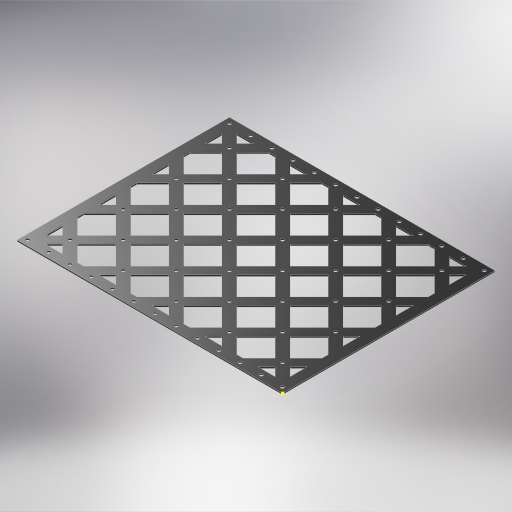
# Autodesk Inventor part: belly pan
Saved by Autodesk Inventor 2024 (Build 280153000, 153)
## iProperties
Created: 2023-12-20
Part Number: belly pan
Material: Generic
Document SubType Name: Modeling
Designer: elite
Density: 1 g/cm^3
Appearance: Glossy - Black
Author: elite
Autodesk Inventor part; units mm, degrees
ref_plane "YZ Plane" through (0, 0, 0) normal (1, 0, 0) x (0, 1, 0)
ref_plane "XZ Plane" through (0, 0, 0) normal (0, 1, 0) x (-1, 0, 0)
ref_plane "XY Plane" through (0, 0, 0) normal (0, 0, 1) x (1, 0, 0)
sketch "Sketch1" plane through (0, 0, 0) normal (0, 1, 0) x (-1, 0, 0)
  line L0 (0, 0) -> (317.5, 0)
  line L1 (317.5, 0) -> (317.5, -254)
  line L2 (317.5, -254) -> (0, -254)
  line L3 (0, -254) -> (0, 0)
  circle A0 centre (311.15, -6.35) radius 2.1082
  circle A1 centre (6.35, -6.35) radius 2.1082
  circle A2 centre (6.35, -247.65) radius 2.1082
  circle A3 centre (311.15, -247.65) radius 2.1082
  line L4 (304.8, -241.3) -> (12.7, -241.3)
  line L5 (12.7, -241.3) -> (12.7, -12.7)
  line L6 (12.7, -12.7) -> (304.8, -12.7)
  line L7 (304.8, -12.7) -> (304.8, -241.3)
  line L8 (304.8, -12.7) -> (76.2, -241.3)
  line L9 (304.8, -241.3) -> (76.2, -12.7)
  line L10 (12.7, -241.3) -> (241.3, -12.7)
  line L11 (6.35, -6.35) -> (241.3, -241.3)
  line L12 (295.8197, -12.7) -> (67.2197, -241.3)
  line L13 (304.8, -21.6803) -> (85.1803, -241.3)
  line L14 (304.8, -232.3197) -> (85.1803, -12.7)
  line L15 (295.8197, -241.3) -> (67.2197, -12.7)
  line L16 (10.8401, -1.8599) -> (250.2803, -241.3)
  line L17 (1.8599, -10.8401) -> (232.3197, -241.3)
  line L18 (12.7, -232.3197) -> (232.3197, -12.7)
  line L19 (21.6803, -241.3) -> (250.2803, -12.7)
  line L20 (368.3, -241.3) -> (139.7, -12.7)
  line L21 (359.3197, -241.3) -> (130.7197, -12.7)
  line L22 (368.3, -232.3197) -> (148.6803, -12.7)
  line L23 (431.8, -241.3) -> (203.2, -12.7)
  line L24 (422.8197, -241.3) -> (194.2197, -12.7)
  line L25 (431.8, -232.3197) -> (212.1803, -12.7)
  line L26 (495.3, -241.3) -> (266.7, -12.7)
  line L27 (486.3197, -241.3) -> (257.7197, -12.7)
  line L28 (495.3, -232.3197) -> (275.6803, -12.7)
  line L29 (241.3, -241.3) -> (12.7, -12.7)
  line L30 (232.3197, -241.3) -> (3.7197, -12.7)
  line L31 (241.3, -232.3197) -> (21.6803, -12.7)
  line L32 (304.8, -241.3) -> (76.2, -12.7)
  line L33 (295.8197, -241.3) -> (67.2197, -12.7)
  line L34 (304.8, -232.3197) -> (85.1803, -12.7)
  line L35 (368.3, -241.3) -> (139.7, -12.7)
  line L36 (359.3197, -241.3) -> (130.7197, -12.7)
  line L37 (368.3, -232.3197) -> (148.6803, -12.7)
  line L38 (431.8, -241.3) -> (203.2, -12.7)
  line L39 (422.8197, -241.3) -> (194.2197, -12.7)
  line L40 (431.8, -232.3197) -> (212.1803, -12.7)
  line L41 (177.8, -241.3) -> (-50.8, -12.7)
  line L42 (168.8197, -241.3) -> (-59.7803, -12.7)
  line L43 (177.8, -232.3197) -> (-41.8197, -12.7)
  line L44 (241.3, -241.3) -> (12.7, -12.7)
  line L45 (232.3197, -241.3) -> (3.7197, -12.7)
  line L46 (241.3, -232.3197) -> (21.6803, -12.7)
  line L47 (304.8, -241.3) -> (76.2, -12.7)
  line L48 (295.8197, -241.3) -> (67.2197, -12.7)
  line L49 (304.8, -232.3197) -> (85.1803, -12.7)
  line L50 (368.3, -241.3) -> (139.7, -12.7)
  line L51 (359.3197, -241.3) -> (130.7197, -12.7)
  line L52 (368.3, -232.3197) -> (148.6803, -12.7)
  line L53 (114.3, -241.3) -> (-114.3, -12.7)
  line L54 (105.3197, -241.3) -> (-123.2803, -12.7)
  line L55 (114.3, -232.3197) -> (-105.3197, -12.7)
  line L56 (177.8, -241.3) -> (-50.8, -12.7)
  line L57 (168.8197, -241.3) -> (-59.7803, -12.7)
  line L58 (177.8, -232.3197) -> (-41.8197, -12.7)
  line L59 (241.3, -241.3) -> (12.7, -12.7)
  line L60 (232.3197, -241.3) -> (3.7197, -12.7)
  line L61 (241.3, -232.3197) -> (21.6803, -12.7)
  line L62 (304.8, -241.3) -> (76.2, -12.7)
  line L63 (295.8197, -241.3) -> (67.2197, -12.7)
  line L64 (304.8, -232.3197) -> (85.1803, -12.7)
  line L65 (50.8, -241.3) -> (-177.8, -12.7)
  line L66 (41.8197, -241.3) -> (-186.7803, -12.7)
  line L67 (50.8, -232.3197) -> (-168.8197, -12.7)
  line L68 (114.3, -241.3) -> (-114.3, -12.7)
  line L69 (105.3197, -241.3) -> (-123.2803, -12.7)
  line L70 (114.3, -232.3197) -> (-105.3197, -12.7)
  line L71 (177.8, -241.3) -> (-50.8, -12.7)
  line L72 (168.8197, -241.3) -> (-59.7803, -12.7)
  line L73 (177.8, -232.3197) -> (-41.8197, -12.7)
  line L74 (241.3, -241.3) -> (12.7, -12.7)
  line L75 (232.3197, -241.3) -> (3.7197, -12.7)
  line L76 (241.3, -232.3197) -> (21.6803, -12.7)
  line L77 (177.8, -232.3197) -> (186.7803, -241.3)
  line L78 (114.3, -232.3197) -> (123.2803, -241.3)
  line L79 (50.8, -232.3197) -> (59.7803, -241.3)
  line L80 (85.1803, -241.3) -> (313.7803, -12.7)
  line L81 (76.2, -232.3197) -> (295.8197, -12.7)
  line L82 (76.2, -241.3) -> (304.8, -12.7)
  line L83 (148.6803, -241.3) -> (377.2803, -12.7)
  line L84 (139.7, -232.3197) -> (359.3197, -12.7)
  line L85 (139.7, -241.3) -> (368.3, -12.7)
  line L86 (212.1803, -241.3) -> (440.7803, -12.7)
  line L87 (203.2, -232.3197) -> (422.8197, -12.7)
  line L88 (203.2, -241.3) -> (431.8, -12.7)
  line L89 (275.6803, -241.3) -> (504.2803, -12.7)
  line L90 (266.7, -232.3197) -> (486.3197, -12.7)
  line L91 (266.7, -241.3) -> (495.3, -12.7)
  line L92 (-41.8197, -241.3) -> (186.7803, -12.7)
  line L93 (-50.8, -232.3197) -> (168.8197, -12.7)
  line L94 (-50.8, -241.3) -> (177.8, -12.7)
  line L95 (21.6803, -241.3) -> (250.2803, -12.7)
  line L96 (12.7, -232.3197) -> (232.3197, -12.7)
  line L97 (12.7, -241.3) -> (241.3, -12.7)
  line L98 (85.1803, -241.3) -> (313.7803, -12.7)
  line L99 (76.2, -232.3197) -> (295.8197, -12.7)
  line L100 (76.2, -241.3) -> (304.8, -12.7)
  line L101 (148.6803, -241.3) -> (377.2803, -12.7)
  line L102 (139.7, -232.3197) -> (359.3197, -12.7)
  line L103 (139.7, -241.3) -> (368.3, -12.7)
  line L104 (212.1803, -241.3) -> (440.7803, -12.7)
  line L105 (203.2, -232.3197) -> (422.8197, -12.7)
  line L106 (203.2, -241.3) -> (431.8, -12.7)
  line L107 (-105.3197, -241.3) -> (123.2803, -12.7)
  line L108 (-114.3, -232.3197) -> (105.3197, -12.7)
  line L109 (-114.3, -241.3) -> (114.3, -12.7)
  line L110 (-41.8197, -241.3) -> (186.7803, -12.7)
  line L111 (-50.8, -232.3197) -> (168.8197, -12.7)
  line L112 (-50.8, -241.3) -> (177.8, -12.7)
  line L113 (21.6803, -241.3) -> (250.2803, -12.7)
  line L114 (12.7, -232.3197) -> (232.3197, -12.7)
  line L115 (12.7, -241.3) -> (241.3, -12.7)
  line L116 (85.1803, -241.3) -> (313.7803, -12.7)
  line L117 (76.2, -232.3197) -> (295.8197, -12.7)
  line L118 (76.2, -241.3) -> (304.8, -12.7)
  line L119 (148.6803, -241.3) -> (377.2803, -12.7)
  line L120 (139.7, -232.3197) -> (359.3197, -12.7)
  line L121 (139.7, -241.3) -> (368.3, -12.7)
  line L122 (-168.8197, -241.3) -> (59.7803, -12.7)
  line L123 (-177.8, -232.3197) -> (41.8197, -12.7)
  line L124 (-177.8, -241.3) -> (50.8, -12.7)
  line L125 (-105.3197, -241.3) -> (123.2803, -12.7)
  line L126 (-114.3, -232.3197) -> (105.3197, -12.7)
  line L127 (-114.3, -241.3) -> (114.3, -12.7)
  line L128 (-41.8197, -241.3) -> (186.7803, -12.7)
  line L129 (-50.8, -232.3197) -> (168.8197, -12.7)
  line L130 (-50.8, -241.3) -> (177.8, -12.7)
  line L131 (21.6803, -241.3) -> (250.2803, -12.7)
  line L132 (12.7, -232.3197) -> (232.3197, -12.7)
  line L133 (12.7, -241.3) -> (241.3, -12.7)
  line L134 (85.1803, -241.3) -> (313.7803, -12.7)
  line L135 (76.2, -232.3197) -> (295.8197, -12.7)
  line L136 (76.2, -241.3) -> (304.8, -12.7)
  line L137 (139.7, -232.3197) -> (130.7197, -241.3)
  line L138 (203.2, -232.3197) -> (194.2197, -241.3)
  line L139 (266.7, -232.3197) -> (257.7197, -241.3)
  point P0 (304.8, -59.7803)
  point P1 (257.7197, -12.7)
  point P2 (276.7697, -31.75)
  point P3 (254, -54.5197)
  point P4 (262.9803, -63.5)
  point P5 (285.75, -40.7303)
  point P6 (285.75, -22.7697)
  point P7 (275.6803, -12.7)
  point P8 (304.8, -41.8197)
  point P9 (294.7303, -31.75)
  point P10 (231.2303, -95.25)
  point P11 (254, -72.4803)
  point P12 (276.7697, -95.25)
  point P13 (254, -118.0197)
  point P14 (222.25, -104.2303)
  point P15 (245.0197, -127)
  point P16 (222.25, -149.7697)
  point P17 (226.7401, -154.2599)
  point P18 (249.5099, -131.4901)
  point P19 (276.7697, -158.75)
  point P20 (254, -181.5197)
  point P21 (258.4901, -186.0099)
  point P22 (281.2599, -163.2401)
  point P23 (304.8, -186.7803)
  point P24 (304.8, -168.8197)
  point P25 (294.7303, -158.75)
  point P26 (304.8, -148.6803)
  point P27 (304.8, -130.7197)
  point P28 (285.75, -149.7697)
  point P29 (262.9803, -127)
  point P30 (285.75, -104.2303)
  point P31 (304.8, -123.2803)
  point P32 (304.8, -105.3197)
  point P33 (294.7303, -95.25)
  point P34 (304.8, -85.1803)
  point P35 (304.8, -67.2197)
  point P36 (285.75, -86.2697)
  point P37 (231.2303, -31.75)
  point P38 (222.25, -22.7697)
  point P39 (212.1803, -12.7)
  point P40 (194.2197, -12.7)
  point P41 (213.2697, -31.75)
  point P42 (190.5, -54.5197)
  point P43 (167.7303, -31.75)
  point P44 (186.7803, -12.7)
  point P45 (168.8197, -12.7)
  point P46 (158.75, -22.7697)
  point P47 (148.6803, -12.7)
  point P48 (130.7197, -12.7)
  point P49 (213.2697, -95.25)
  point P50 (190.5, -118.0197)
  point P51 (199.4803, -127)
  point P52 (222.25, -86.2697)
  point P53 (199.4803, -63.5)
  point P54 (222.25, -40.7303)
  point P55 (245.0197, -63.5)
  point P56 (222.25, -167.7303)
  point P57 (245.0197, -190.5)
  point P58 (222.25, -213.2697)
  point P59 (199.4803, -190.5)
  point P60 (158.75, -231.2303)
  point P61 (167.7303, -222.25)
  point P62 (190.5, -199.4803)
  point P63 (213.2697, -222.25)
  point P64 (222.25, -231.2303)
  point P65 (231.2303, -222.25)
  point P66 (254, -199.4803)
  point P67 (276.7697, -222.25)
  point P68 (285.75, -231.2303)
  point P69 (294.7303, -222.25)
  point P70 (304.8, -212.1803)
  point P71 (304.8, -194.2197)
  point P72 (285.75, -213.2697)
  point P73 (262.9803, -190.5)
  point P74 (285.75, -167.7303)
  point P75 (231.2303, -158.75)
  point P76 (254, -135.9803)
  point P77 (40.7303, -222.25)
  point P78 (31.75, -231.2303)
  point P79 (190.5, -135.9803)
  point P80 (213.2697, -158.75)
  point P81 (167.7303, -95.25)
  point P82 (158.75, -104.2303)
  point P83 (181.5197, -127)
  point P84 (158.75, -149.7697)
  point P85 (135.9803, -127)
  point P86 (127, -135.9803)
  point P87 (149.7697, -158.75)
  point P88 (127, -181.5197)
  point P89 (104.2303, -158.75)
  point P90 (95.25, -167.7303)
  point P91 (118.0197, -190.5)
  point P92 (95.25, -213.2697)
  point P93 (72.4803, -190.5)
  point P94 (63.5, -199.4803)
  point P95 (86.2697, -222.25)
  point P96 (95.25, -231.2303)
  point P97 (104.2303, -222.25)
  point P98 (127, -199.4803)
  point P99 (149.7697, -222.25)
  point P100 (158.75, -213.2697)
  point P101 (135.9803, -190.5)
  point P102 (158.75, -167.7303)
  point P103 (181.5197, -190.5)
  point P104 (190.5, -181.5197)
  point P105 (167.7303, -158.75)
  point P106 (158.75, -86.2697)
  point P107 (135.9803, -63.5)
  point P108 (127, -72.4803)
  point P109 (149.7697, -95.25)
  point P110 (127, -118.0197)
  point P111 (104.2303, -95.25)
  point P112 (95.25, -104.2303)
  point P113 (118.0197, -127)
  point P114 (95.25, -149.7697)
  point P115 (72.4803, -127)
  point P116 (63.5, -135.9803)
  point P117 (86.2697, -158.75)
  point P118 (63.5, -181.5197)
  point P119 (40.7303, -158.75)
  point P120 (31.75, -167.7303)
  point P121 (54.5197, -190.5)
  point P122 (31.75, -213.2697)
  point P123 (12.7, -194.2197)
  point P124 (12.7, -212.1803)
  point P125 (22.7697, -222.25)
  point P126 (190.5, -72.4803)
  point P127 (181.5197, -63.5)
  point P128 (86.2697, -95.25)
  point P129 (63.5, -118.0197)
  point P130 (40.7303, -95.25)
  point P131 (63.5, -72.4803)
  point P132 (118.0197, -63.5)
  point P133 (95.25, -86.2697)
  point P134 (72.4803, -63.5)
  point P135 (95.25, -40.7303)
  point P136 (158.75, -40.7303)
  point P137 (149.7697, -31.75)
  point P138 (127, -54.5197)
  point P139 (104.2303, -31.75)
  point P140 (123.2803, -12.7)
  point P141 (105.3197, -12.7)
  point P142 (95.25, -22.7697)
  point P143 (86.2697, -31.75)
  point P144 (63.5, -54.5197)
  point P145 (40.7303, -31.75)
  point P146 (59.7803, -12.7)
  point P147 (41.8197, -12.7)
  point P148 (31.75, -22.7697)
  point P149 (21.6803, -12.7)
  point P150 (12.7, -21.6803)
  point P151 (22.7697, -31.75)
  point P152 (12.7, -41.8197)
  point P153 (12.7, -59.7803)
  point P154 (31.75, -40.7303)
  point P155 (54.5197, -63.5)
  point P156 (31.75, -86.2697)
  point P157 (12.7, -67.2197)
  point P158 (12.7, -85.1803)
  point P159 (22.7697, -95.25)
  point P160 (12.7, -105.3197)
  point P161 (12.7, -123.2803)
  point P162 (31.75, -104.2303)
  point P163 (54.5197, -127)
  point P164 (31.75, -149.7697)
  point P165 (12.7, -130.7197)
  point P166 (12.7, -148.6803)
  point P167 (22.7697, -158.75)
  point P168 (12.7, -168.8197)
  point P169 (12.7, -186.7803)
  dimension "d60" = 317.5
  dimension "d61" = 254
  dimension "d62" = 4.2164
  dimension "d63" = 6.35
  dimension "d64" = 6.35
  dimension "d65" = 4.2164
  dimension "d66" = 6.35
  dimension "d69" = 241.3
  dimension "d74" = 6.35
  dimension "d75" = 12.7
  dimension "d76" = 12.7
  dimension "d77" = 12.7
  dimension "d78" = 12.7
  dimension "d79" = 45
  dimension "d80" = 45
  dimension "d81" = 45
  dimension "d82" = 45
  dimension "d83" = 6.35
  dimension "d84" = 6.35
  dimension "d85" = 6.35
  dimension "d86" = 6.35
  dimension "d87" = 6.35
  dimension "d88" = 6.35
  dimension "d89" = 6.35
  dimension "d90" = 6.35
  dimension "d93" = 63.5
  dimension "d96" = 63.5
  dimension "d101" = 63.5
  dimension "d104" = 63.5
  constraints: 276 end point, 228 horizontal alignment, 128 parallel, 4 centre point, 4 point on line, 2 vertical, 1 horizontal, 1 perpendicular, 30 other
  measures "d60" distance of L1.end L2.end
  measures "d61" distance of L0.end L1.end
  measures "d62" diameter of A0
  measures "d63" distance from line of L0 A0.centre
  measures "d64" distance from line of L1 A0.centre
  measures "d65" diameter of A1
  measures "d66" distance from line of L3 L11.start
  measures "d69" distance of L11.start A2.centre
  measures "d74" distance from line of L0 L11.start
  measures "d76" distance between parallel lines of L1 L7
  measures "d78" distance between parallel lines of L3 L5
  measures "d79" angle to the sketch x axis of L8
  measures "d80" angle of L7 L9
  measures "d81" angle of L5 L10
  measures "d82" angle of L5 L11
  measures "d83" distance between parallel lines of L8 L12
  measures "d84" distance between parallel lines of L8 L13
  measures "d85" distance between parallel lines of L9 L14
  measures "d86" distance between parallel lines of L9 L15
  measures "d87" distance between parallel lines of L11 L16
  measures "d88" distance between parallel lines of L11 L17
  measures "d89" distance between parallel lines of L10 L18
  measures "d90" distance between parallel lines of L10 L19
  measures "d93" distance of L7.end L20.start
  measures "d96" distance of L7.end L29.start
  measures "d101" distance of L19.start L80.start
  measures "d104" distance of L19.start L92.start
extrude "Extrusion1" add sketch "Sketch1" along normal blind 1.5875 contours L0 L1 L28 L7 L6 L5 L123 L3 | L43 L124 L3 | L123 L5 L124 L43 | L84 L26 L7 L28 | L1 L26 L84 | L41 L122 L3 | L124 L43 L122 L41 | L124 L5 L122 L43 | L123 L17 L124 L5 | L85 L27 L84 L26 | L1 L27 L85 | L7 L26 L13 L28 | L84 L27 L7 L26 | L42 L5 L108 L3 | L122 L41 L5 L42 | L122 L43 L5 L41 | L122 L5 L43 | L124 L17 L122 L5 | L5 L11 L123 L17 | L123 L11 L124 L17 | L83 L7 L85 L27 | L1 L25 L7 L83 | L85 L7 L84 L27 | L13 L28 L8 L7 | L7 L27 L13 L26 | L13 L26 L8 L28 | L84 L7 L27 | L55 L109 L3 | L108 L5 L109 L55 | L5 L41 L108 L42 | L5 L43 L108 L41 | L124 L11 L122 L17 | L6 L16 L123 L11 | L123 L16 L124 L11 | L87 L23 L7 L25 | L1 L23 L87 | L83 L25 L85 L7 | L85 L25 L84 L7 | L8 L28 L12 L6 | L13 L27 L8 L26 | L8 L26 L12 L28 | L53 L107 L3 | L109 L55 L107 L53 | L109 L5 L107 L55 | L108 L42 L109 L5 | L108 L41 L109 L42 | L108 L43 L109 L41 | L108 L17 L109 L43 | L122 L11 L108 L17 | L124 L16 L122 L11 | L123 L6 L124 L16 | L88 L24 L87 L23 | L1 L24 L88 | L7 L23 L83 L25 | L87 L24 L7 L23 | L83 L23 L85 L25 | L85 L23 L84 L25 | L13 L25 L8 L27 | L8 L27 L12 L26 | L12 L26 L6 L28 | L84 L23 L13 L25 | L54 L5 L93 L3 | L107 L53 L5 L54 | L107 L55 L5 L53 | L107 L5 L55 | L109 L42 L107 L5 | L109 L41 L107 L42 | L109 L43 L107 L41 | L109 L17 L107 L43 | L108 L11 L109 L17 | L122 L16 L108 L11 | L124 L6 L122 L16 | L86 L7 L88 L24 | L1 L22 L7 L86 | L88 L7 L87 L24 | L7 L24 L83 L23 | L87 L7 L24 | L83 L24 L85 L23 | L85 L24 L84 L23 | L13 L23 L8 L25 | L8 L25 L12 L27 | L12 L27 L6 L26 | L84 L24 L13 L23 | L67 L94 L3 | L93 L5 L94 L67 | L5 L53 L93 L54 | L5 L55 L93 L53 | L107 L41 L93 L42 | L107 L43 L93 L41 | L109 L11 L107 L17 | L108 L16 L109 L11 | L90 L20 L7 L22 | L1 L20 L90 | L86 L22 L88 L7 | L88 L22 L87 L7 | L83 L22 L85 L24 | L85 L22 L84 L24 | L13 L24 L8 L23 | L8 L23 L12 L25 | L65 L92 L3 | L94 L67 L92 L65 | L94 L5 L92 L67 | L93 L54 L94 L5 | L93 L53 L94 L54 | L93 L55 L94 L53 | L93 L42 L94 L55 | L93 L41 L94 L42 | L93 L43 L94 L41 | L93 L17 L94 L43 | L107 L11 L93 L17 | L109 L16 L107 L11 | L108 L15 L109 L16 | L91 L21 L90 L20 | L1 L21 L91 | L7 L20 L86 L22 | L90 L21 L7 L20 | L86 L20 L88 L22 | L88 L20 L87 L22 | L87 L20 L83 L22 | L83 L20 L85 L22 | L85 L20 L84 L22 | L13 L22 L8 L24 | L8 L24 L12 L23 | L12 L23 L19 L25 | L84 L20 L13 L22 | L66 L5 L4 L7 L89 L1 L2 L3 | L92 L65 L5 L66 | L92 L67 L5 L65 | L92 L5 L67 | L94 L54 L92 L5 | L94 L53 L92 L54 | L94 L55 L92 L53 | L94 L42 L92 L55 | L94 L41 L92 L42 | L94 L43 L92 L41 | L94 L17 L92 L43 | L93 L11 L94 L17 | L107 L16 L93 L11 | L109 L15 L107 L16 | L108 L9 L109 L15 | L15 L6 L9 L108 | L89 L7 L91 L21 | L91 L7 L90 L21 | L7 L21 L86 L20 | L90 L7 L21 | L86 L21 L88 L20 | L88 L21 L87 L20 | L87 L21 L83 L20 | L83 L21 L85 L20 | L85 L21 L84 L20 | L19 L25 L10 L6 | L13 L20 L8 L22 | L8 L22 L12 L24 | L12 L24 L19 L23 | L19 L23 L10 L25 | L84 L21 L13 L20 | L5 L65 L18 L66 | L5 L67 L18 L65 | L92 L53 L18 L54 | L92 L55 L18 L53 | L92 L41 L18 L42 | L92 L43 L18 L41 | L94 L11 L92 L17 | L93 L16 L94 L11 | L109 L9 L107 L15 | L108 L14 L109 L9 | L9 L6 L14 L108 | L89 L14 L91 L7 | L91 L14 L90 L7 | L86 L14 L88 L21 | L88 L14 L87 L21 | L83 L14 L85 L21 | L85 L14 L84 L21 | L10 L25 L18 L6 | L13 L21 L8 L20 | L8 L20 L12 L22 | L19 L24 L10 L23 | L10 L23 L18 L25 | L18 L66 L10 L5 | L18 L65 L10 L66 | L18 L67 L10 L65 | L18 L54 L10 L67 | L18 L53 L10 L54 | L18 L55 L10 L53 | L18 L42 L10 L55 | L18 L41 L10 L42 | L18 L43 L10 L41 | L18 L17 L10 L43 | L92 L11 L18 L17 | L94 L16 L92 L11 | L93 L15 L94 L16 | L107 L9 L93 L15 | L109 L14 L107 L9 | L108 L6 L109 L14 | L7 L9 L89 L14 | L89 L9 L91 L14 | L91 L9 L90 L14 | L90 L9 L86 L14 | L86 L9 L88 L14 | L88 L9 L87 L14 | L87 L9 L83 L14 | L83 L9 L85 L14 | L85 L9 L84 L14 | L13 L14 L8 L21 | L8 L21 L12 L20 | L12 L20 L19 L22 | L19 L22 L10 L24 | L10 L24 L18 L23 | L18 L23 L6 L25 | L84 L9 L13 L14 | L10 L66 L19 L4 | L10 L65 L19 L66 | L10 L67 L19 L65 | L10 L54 L19 L67 | L10 L53 L19 L54 | L10 L55 L19 L53 | L10 L42 L19 L55 | L10 L41 L19 L42 | L10 L43 L19 L41 | L18 L11 L10 L17 | L10 L17 L19 L43 | L92 L16 L18 L11 | L94 L15 L92 L16 | L93 L9 L94 L15 | L107 L14 L93 L9 | L109 L6 L107 L14 | L4 L15 L89 L9 | L89 L15 L91 L9 | L91 L15 L90 L9 | L90 L15 L86 L9 | L86 L15 L88 L9 | L88 L15 L87 L9 | L87 L15 L83 L9 | L83 L15 L85 L9 | L85 L15 L84 L9 | L13 L9 L8 L14 | L8 L14 L12 L21 | L12 L21 L19 L20 | L19 L20 L10 L22 | L10 L22 L18 L24 | L18 L24 L6 L23 | L84 L15 L13 L9 | L19 L65 L4 L66 | L19 L67 L79 L4 L65 | L19 L53 L12 L54 | L19 L55 L12 L53 | L19 L41 L12 L42 | L19 L43 L12 L41 | L10 L11 L19 L17 | L18 L16 L10 L11 | L94 L9 L92 L15 | L93 L14 L94 L9 | L89 L4 L91 L15 | L91 L4 L139 L90 L15 | L86 L16 L88 L15 | L88 L16 L87 L15 | L83 L16 L85 L15 | L85 L16 L84 L15 | L13 L15 L8 L9 | L8 L9 L12 L14 | L19 L21 L10 L20 | L10 L20 L18 L22 | L54 L8 L4 L12 | L12 L53 L8 L54 | L12 L55 L8 L53 | L12 L42 L8 L55 | L12 L41 L8 L42 | L12 L43 L8 L41 | L10 L16 L19 L11 | L19 L11 L12 L17 | L18 L15 L10 L16 | L12 L17 L8 L43 | L92 L9 L18 L15 | L94 L14 L92 L9 | L93 L21 L94 L14 | L86 L11 L88 L16 | L16 L4 L11 L86 | L88 L11 L87 L16 | L87 L11 L83 L16 | L83 L11 L85 L16 | L85 L11 L84 L16 | L8 L15 L12 L9 | L13 L16 L8 L15 | L12 L9 L19 L14 | L19 L14 L10 L21 | L10 L21 L18 L20 | L18 L20 L92 L22 | L84 L11 L13 L16 | L54 L13 L4 L8 | L8 L53 L13 L54 | L8 L55 L13 L53 | L8 L42 L13 L55 | L8 L41 L13 L42 | L8 L43 L13 L41 | L10 L15 L19 L16 | L19 L16 L12 L11 | L12 L11 L8 L17 | L18 L9 L10 L15 | L8 L17 L13 L43 | L92 L14 L18 L9 | L94 L21 L92 L14 | L93 L20 L94 L21 | L21 L6 L20 L93 | L86 L17 L88 L11 | L11 L4 L17 L86 | L88 L17 L87 L11 | L87 L17 L83 L11 | L83 L17 L85 L11 | L85 L17 L84 L11 | L92 L22 L94 L6 | L8 L16 L12 L15 | L12 L15 L19 L9 | L13 L11 L8 L16 | L19 L9 L10 L14 | L10 L14 L18 L21 | L18 L21 L92 L20 | L92 L20 L94 L22 | L84 L17 L13 L11 | L13 L53 L4 L54 | L13 L55 L78 L4 L53 | L13 L41 L84 L42 | L13 L43 L84 L41 | L10 L9 L19 L15 | L12 L16 L8 L11 | L8 L11 L13 L17 | L18 L14 L10 L9 | L94 L20 L92 L21 | L93 L22 L94 L20 | L20 L6 L22 L93 | L86 L4 L88 L17 | L88 L4 L138 L87 L17 | L83 L43 L85 L17 | L85 L43 L84 L17 | L94 L22 L93 L6 | L84 L41 L85 L42 | L42 L85 L4 L137 L84 | L84 L43 L85 L41 | L83 L41 L85 L43 | L43 L77 L4 L41 L83 | L85 L41 L83 L42 | L42 L83 L4 L85 | L41 L4 L42 L83
sketch "Sketch3" plane through (0, 1.5875, 0) normal (0, 1, 0) x (1, 0, 0)
  circle A0 centre (-311.15, 6.35) radius 2.1082 projected
  line L0 (-317.5, 0) -> (0, 0) projected
  circle A1 centre (-311.15, 247.65) radius 2.1082 projected
  line L1 (0, 254) -> (-317.5, 254) projected
  circle A2 centre (-311.15, 247.65) radius 2.1082
  circle A3 centre (-311.15, 6.35) radius 2.1082
  circle A4 centre (-285.75, 6.35) radius 2.1082
  circle A5 centre (-285.75, 247.65) radius 2.1082
  circle A6 centre (-260.35, 6.35) radius 2.1082
  circle A7 centre (-260.35, 247.65) radius 2.1082
  circle A8 centre (-234.95, 6.35) radius 2.1082
  circle A9 centre (-234.95, 247.65) radius 2.1082
  circle A10 centre (-209.55, 6.35) radius 2.1082
  circle A11 centre (-209.55, 247.65) radius 2.1082
  circle A12 centre (-184.15, 6.35) radius 2.1082
  circle A13 centre (-184.15, 247.65) radius 2.1082
  circle A14 centre (-158.75, 6.35) radius 2.1082
  circle A15 centre (-158.75, 247.65) radius 2.1082
  circle A16 centre (-133.35, 6.35) radius 2.1082
  circle A17 centre (-133.35, 247.65) radius 2.1082
  circle A18 centre (-107.95, 6.35) radius 2.1082
  circle A19 centre (-107.95, 247.65) radius 2.1082
  circle A20 centre (-82.55, 6.35) radius 2.1082
  circle A21 centre (-82.55, 247.65) radius 2.1082
  circle A22 centre (-57.15, 6.35) radius 2.1082
  circle A23 centre (-57.15, 247.65) radius 2.1082
  circle A24 centre (-31.75, 6.35) radius 2.1082
  circle A25 centre (-31.75, 247.65) radius 2.1082
  circle A26 centre (-6.35, 6.35) radius 2.1082
  circle A27 centre (-6.35, 247.65) radius 2.1082
  circle A28 centre (19.05, 6.35) radius 2.1082
  circle A29 centre (19.05, 247.65) radius 2.1082
  dimension "d109" = 25.4
  constraints: 28 centre point, 2 coincident, 2 concentric, 1 horizontal, 52 other
  measures "d109" distance of A3.centre A4.centre
extrude "Extrusion3" cut sketch "Sketch3" against normal blind 317.5
sketch "Sketch4" plane through (0, 1.5875, 0) normal (0, 1, 0) x (1, 0, 0)
  point P0 (0, 0)
sketch "Sketch5" plane through (0, 1.5875, 0) normal (0, 1, 0) x (1, 0, 0)
  line L0 (-285.75, 22.7697) -> (-275.6803, 12.7) projected
  line L1 (-285.75, 40.7303) -> (-285.75, 22.7697)
  circle A0 centre (-285.75, 31.75) radius 2.1082
  line L2 (-317.5, 254) -> (-317.5, 0) projected
  line L3 (-317.5, 0) -> (0, 0) projected
  circle A1 centre (-222.25, 31.75) radius 2.1082
  circle A2 centre (-158.75, 31.75) radius 2.1082
  circle A3 centre (-95.25, 31.75) radius 2.1082
  circle A4 centre (-31.75, 31.75) radius 2.1082
  circle A5 centre (-285.75, 95.25) radius 2.1082
  circle A6 centre (-222.25, 95.25) radius 2.1082
  circle A7 centre (-158.75, 95.25) radius 2.1082
  circle A8 centre (-95.25, 95.25) radius 2.1082
  circle A9 centre (-31.75, 95.25) radius 2.1082
  circle A10 centre (-285.75, 158.75) radius 2.1082
  circle A11 centre (-222.25, 158.75) radius 2.1082
  circle A12 centre (-158.75, 158.75) radius 2.1082
  circle A13 centre (-95.25, 158.75) radius 2.1082
  circle A14 centre (-31.75, 158.75) radius 2.1082
  circle A15 centre (-285.75, 222.25) radius 2.1082
  circle A16 centre (-222.25, 222.25) radius 2.1082
  circle A17 centre (-158.75, 222.25) radius 2.1082
  circle A18 centre (-95.25, 222.25) radius 2.1082
  circle A19 centre (-31.75, 222.25) radius 2.1082
  line L4 (-254, 199.4803) -> (-254, 181.5197)
  circle A20 centre (-254, 190.5) radius 2.1082
  circle A21 centre (-254, 127) radius 2.1082
  circle A22 centre (-254, 63.5) radius 2.1082
  circle A23 centre (-190.5, 190.5) radius 2.1082
  circle A24 centre (-190.5, 127) radius 2.1082
  circle A25 centre (-190.5, 63.5) radius 2.1082
  circle A26 centre (-127, 190.5) radius 2.1082
  circle A27 centre (-127, 127) radius 2.1082
  circle A28 centre (-127, 63.5) radius 2.1082
  circle A29 centre (-63.5, 190.5) radius 2.1082
  circle A30 centre (-63.5, 127) radius 2.1082
  circle A31 centre (-63.5, 63.5) radius 2.1082
  dimension "d116" = 4.2164
  dimension "d119" = 63.5
  dimension "d122" = 63.5
  dimension "d125" = 4.2164
  dimension "d128" = 63.5
  dimension "d131" = 63.5
  constraints: 32 centre point, 4 end point, 3 vertical, 2 horizontal, 2 midpoint, 60 other
  measures "d116" diameter of A0
  measures "d119" distance of A0.centre A1.centre
  measures "d122" distance of A0.centre A5.centre
  measures "d125" diameter of A20
  measures "d128" distance of A20.centre A21.centre
  measures "d131" distance of A20.centre A23.centre
extrude "Extrusion4" cut sketch "Sketch5" against normal blind 1.5875
body "Solid1"
